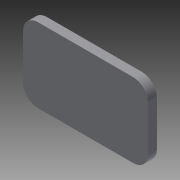
# Autodesk Inventor part: Bottom Block
Saved by Autodesk Inventor 2013 SP1 (Build 170176100, 176)
## iProperties
Created: 2013-08-06
Part Number: Bottom Block
Material: Generic
Document SubType Name: Modeling
Designer: Eric
Density: 1 g/cm^3
Author: Eric
Autodesk Inventor part; units mm, degrees
ref_plane "YZ Plane" through (0, 0, 0) normal (1, 0, 0) x (0, 1, 0)
ref_plane "XZ Plane" through (0, 0, 0) normal (0, 1, 0) x (-1, 0, 0)
ref_plane "XY Plane" through (0, 0, 0) normal (0, 0, 1) x (1, 0, 0)
sketch "Sketch1" plane through (0, 0, 0) normal (0, 1, 0) x (-1, 0, 0)
  line L0 (0, -5) -> (32, -5)
  line L1 (37, 0) -> (37, 15)
  line L2 (32, 20) -> (0, 20)
  line L3 (-5, 15) -> (-5, 0)
  arc A0 (0, 20) -> (-5, 15) centre (0, 15) ccw
  arc A1 (37, 15) -> (32, 20) centre (32, 15) ccw
  arc A2 (32, -5) -> (37, 0) centre (32, 0) ccw
  arc A3 (-5, 0) -> (0, -5) centre (0, 0) ccw
  point P0 (0, 0)
  point P1 (-5, -5)
  point P2 (37, -5)
  point P3 (-5, 20)
  dimension "d0" = 5
  dimension "d1" = 42
  dimension "d2" = 25
  dimension "d3" = 5
  dimension "d4" = 5
  constraints: 8 end point, 8 point on circle, 8 tangent, 6 point on line, 4 centre point, 3 equal radius, 2 parallel, 1 horizontal, 1 perpendicular
  measures "d0" distance from line of L0 point (0, 0)
  measures "d1" distance of point (-5, -5) point (37, -5)
  measures "d2" distance of point (-5, 20) point (-5, -5)
  measures "d3" distance from line of point (0, 0) L3
  measures "d4" radius of A0
extrude "Extrusion1" add sketch "Sketch1" along normal blind 3
body "Solid1"
